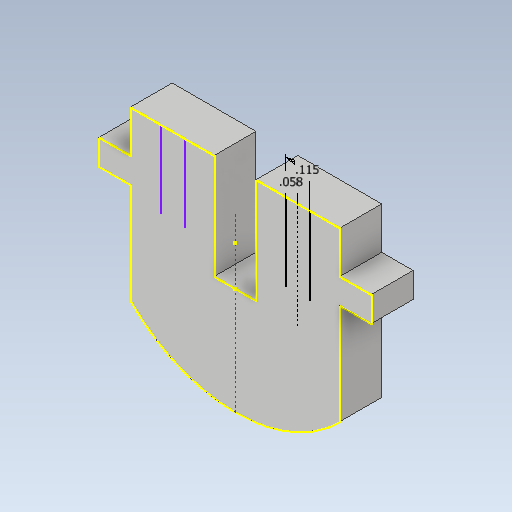
# Autodesk Inventor part: TopPegCor
Saved by Autodesk Inventor 2020.1 (Build 241239000, 239)
## iProperties
Created: 2019-10-24
Part Number: TopPegCor
Material: Generic
Document SubType Name: Modeling
Designer: j8qin
Density: 1 g/cm^3
Appearance: Default
Author: j8qin
Autodesk Inventor part; units mm, degrees
ref_plane "YZ Plane" through (0, 0, 0) normal (1, 0, 0) x (0, 1, 0)
ref_plane "XZ Plane" through (0, 0, 0) normal (0, 1, 0) x (-1, 0, 0)
ref_plane "XY Plane" through (0, 0, 0) normal (0, 0, 1) x (1, 0, 0)
sketch "Sketch1" plane through (0, 0, 0) normal (0, 0, 1) x (1, 0, 0)
  line L0 (-12.7, -7.62) -> (12.7, -7.62) construction
  line L1 (12.7, -7.62) -> (-12.7, 7.62) construction
  line L2 (12.7, 7.62) -> (-12.7, -7.62) construction
  line L3 (-6.35, 0) -> (-6.35, 7.62) construction
  line L4 (6.35, 7.62) -> (-6.35, 0) construction
  line L5 (6.35, 0) -> (-6.35, 7.62) construction
  line L6 (-12.7, 2.667) -> (-16.51, 2.667) construction
  line L7 (-16.51, 4.953) -> (-12.7, 4.953) construction
  line L8 (-8.89, 4.953) -> (-8.89, 2.667) construction
  line L9 (-8.89, 2.667) -> (-16.51, 4.953) construction
  line L10 (-16.51, 2.667) -> (-8.89, 4.953) construction
  line L11 (12.7, 2.667) -> (16.51, 2.667) construction
  line L12 (16.51, 4.953) -> (12.7, 4.953) construction
  line L13 (8.89, 4.953) -> (8.89, 2.667) construction
  line L14 (8.89, 2.667) -> (16.51, 4.953) construction
  line L15 (16.51, 2.667) -> (8.89, 4.953) construction
  line L16 (-19.9417, -12.954) -> (22.1348, -12.954) construction
  arc A0 (-12.7, -7.62) -> (12.7, -7.62) centre (0, 4.832) ccw
  line L17 (12.7, 7.62) -> (6.35, 7.62) construction
  line L18 (-6.35, 7.62) -> (-12.7, 7.62) construction
  line L19 (-12.7, 2.286) -> (-12.7, -7.62)
  line L20 (12.7, -7.62) -> (12.7, 2.286)
  line L21 (-12.7, 7.62) -> (-12.7, 12.7)
  line L22 (-12.7, 12.7) -> (-6.35, 12.7)
  line L23 (-6.35, 12.7) -> (-6.35, 7.62) construction
  line L24 (6.35, 12.7) -> (12.7, 12.7)
  line L25 (12.7, 12.7) -> (12.7, 7.62)
  line L26 (6.35, 12.7) -> (5.715, 12.7)
  line L27 (5.715, 0.381) -> (5.715, 0) construction
  line L28 (-6.35, 12.7) -> (-5.715, 12.7)
  line L29 (-5.715, 0.381) -> (-5.715, 0) construction
  line L30 (6.35, 1.905) -> (6.35, 0) construction
  line L31 (-5.715, 0) -> (-3.175, 0) construction
  line L32 (-3.175, 0) -> (-3.175, 0.9525) construction
  line L33 (5.715, 0) -> (3.175, 0) construction
  line L34 (3.175, 0) -> (3.175, 0.9525) construction
  line L35 (-5.715, 12.7) -> (-3.175, 12.7)
  line L36 (3.175, 12.7) -> (5.715, 12.7)
  line L37 (-2.54, 0) -> (2.54, 0)
  line L38 (-12.7, 7.62) -> (-16.51, 7.62)
  line L39 (-16.51, 7.62) -> (-16.51, 4.572)
  line L40 (-16.51, 4.572) -> (-12.7, 4.572)
  line L41 (-12.7, 4.572) -> (-12.7, 2.286)
  line L42 (12.7, 7.62) -> (16.51, 7.62)
  line L43 (16.51, 7.62) -> (16.51, 4.572)
  line L44 (16.51, 4.572) -> (12.7, 4.572)
  line L45 (12.7, 4.572) -> (12.7, 2.286)
  line L46 (-3.175, 12.7) -> (-2.54, 12.7)
  line L47 (-2.54, 12.7) -> (-2.54, 0)
  line L48 (3.175, 12.7) -> (2.54, 12.7)
  line L49 (2.54, 12.7) -> (2.54, 0)
  line L50 (5.715, 0) -> (3.175, 0) construction
  line L51 (2.54, 0) -> (-5.715, 0) construction
  point P0 (0, 0)
  point P1 (0, 3.81)
  point P2 (-12.7, 3.81)
  point P3 (12.7, 3.81)
  dimension "d0" = 15.24
  dimension "d1" = 25.4
  dimension "d2" = 12.7
  dimension "d5" = 7.62
  dimension "d6" = 2.286
  dimension "d7" = 7.62
  dimension "d8" = 2.286
  dimension "d12" = 5.08
  dimension "d15" = 3.81
  dimension "d20" = 0.635
  dimension "d21" = 0.635
  dimension "d24" = 2.54
  dimension "d25" = 2.54
  dimension "d28" = 3.81
  dimension "d29" = 3.048
  dimension "d32" = 0.635
  constraints: 104 end point, 25 perpendicular, 8 midpoint, 7 point on line, 6 parallel, 5 horizontal, 4 collinear, 3 vertical, 2 point on circle, 1 centre point, 1 tangent
  measures "d0" distance of L0.end L2.start
  measures "d1" distance of L1.end L2.start
  measures "d2" distance of L5.start L3.start
  measures "d5" distance of L8.end L6.end
  measures "d6" distance of L6.end L7.start
  measures "d7" distance of L13.end L11.end
  measures "d8" distance of L12.start L11.end
  measures "d12" distance of L1.end L21.end
  measures "d15" distance from line of L17 point (12.7, 3.81)
  measures "d20" distance of L24.start L26.end
  measures "d21" distance of L22.end L28.end
  measures "d24" distance of L29.end L31.end
  measures "d25" distance of L27.end L33.end
  measures "d28" distance of L1.end L38.end
  measures "d29" distance of L38.end L39.end
  measures "d32" distance of L35.end L46.end
extrude "Extrusion7" add sketch "Sketch1" along normal mid plane 5.08
sketch "Sketch2" plane through (0, 0, 2.54) normal (0, 0, 1) x (1, 0, 0)
  arc A0 (-12.7, -7.62) -> (12.7, -7.62) centre (0, 4.832) ccw projected
  line L0 (12.7, -7.62) -> (12.7, 4.572) projected
  line L1 (12.7, 4.572) -> (16.51, 4.572) projected
  line L2 (16.51, 4.572) -> (16.51, 7.62) projected
  line L3 (16.51, 7.62) -> (12.7, 7.62) projected
  line L4 (12.7, 7.62) -> (12.7, 12.7) projected
  line L5 (12.7, 12.7) -> (2.54, 12.7) projected
  line L6 (2.54, 12.7) -> (2.54, 0) projected
  line L7 (2.54, 0) -> (-2.54, 0) projected
  line L8 (-2.54, 0) -> (-2.54, 12.7) projected
  line L9 (-2.54, 12.7) -> (-12.7, 12.7) projected
  line L10 (-12.7, 12.7) -> (-12.7, 7.62) projected
  line L11 (-12.7, 7.62) -> (-16.51, 7.62) projected
  line L12 (-16.51, 7.62) -> (-16.51, 4.572) projected
  line L13 (-16.51, 4.572) -> (-12.7, 4.572) projected
  line L14 (-12.7, 4.572) -> (-12.7, -7.62) projected
  line L15 (0, 8.0449) -> (0, -12.954) construction
  line L16 (12.7, 12.7) -> (2.54, 12.7) construction
  line L17 (7.62, 12.7) -> (7.62, -0.0804) construction
  line L18 (6.1595, 12.7) -> (6.1595, 3.3381)
  line L19 (9.0805, 12.7) -> (9.0805, 3.3381)
  line L20 (-6.1595, 12.7) -> (-6.1595, 3.3381)
  line L21 (-9.0805, 12.7) -> (-9.0805, 3.3381)
  point P0 (0, 0)
  dimension "d35" = 1.4605
  dimension "d36" = 2.921
  constraints: 12 end point, 4 symmetric about line, 3 vertical, 2 point on line, 1 midpoint, 1 point on circle
  measures "d35" distance between parallel lines of L17 L18
  measures "d36" distance between parallel lines of L18 L19
body "Solid7"
